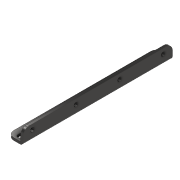
# Autodesk Inventor part: beugel armsteun
Saved by Autodesk Inventor 2020.3 (Build 243373000, 373)
## iProperties
Created: 2020-09-11
Part Number: beugel armsteun
Material: Stainless Steel
Document SubType Name: Modeling
Designer: Svend
Density: 8 g/cm^3
Appearance: Semi-Polished
Author: Svend
Autodesk Inventor part; units mm, degrees
ref_plane "YZ Plane" through (0, 0, 0) normal (1, 0, 0) x (0, 1, 0)
ref_plane "XZ Plane" through (0, 0, 0) normal (0, 1, 0) x (-1, 0, 0)
ref_plane "XY Plane" through (0, 0, 0) normal (0, 0, 1) x (1, 0, 0)
sketch "Sketch1" plane through (0, 0, 0) normal (0, 0, 1) x (1, 0, 0)
  line L0 (0, 0) -> (-25, 0)
  line L1 (-25, 0) -> (-25, 4)
  line L2 (-25, 4) -> (-4, 4)
  line L3 (-4, 4) -> (-4, 23)
  line L4 (-4, 23) -> (0, 23)
  line L5 (0, 23) -> (0, 0)
  dimension "d0" = 25
  dimension "d1" = 4
  dimension "d2" = 23
  constraints: 12 end point, 4 perpendicular, 3 horizontal
  measures "d0" distance of L0.start L0.end
  measures "d1" distance of L0.end L1.end
  measures "d2" distance of L4.end L0.start
extrude "Extrusion1" add sketch "Sketch1" along normal mid plane 240
sketch "Sketch2" plane through (-4, 4, 120) normal (-1, 0, 0) x (0, 0, 1)
  circle A0 centre (-225, 11) radius 3.5
  line L0 (-240, 0) -> (-240, 19) projected
  line L1 (-240, 19) -> (0, 19) projected
  circle A1 centre (-155, 11) radius 3.5
  circle A2 centre (-85, 11) radius 3.5
  circle A3 centre (-15, 11) radius 3.5
  line L2 (0, 19) -> (0, 0) projected
  point P0 (-120, -4)
  dimension "d5" = 7
  dimension "d6" = 15
  dimension "d7" = 8
  dimension "d8" = 15
  dimension "d9" = 70
  dimension "d10" = 70
  constraints: 4 centre point, 3 equal radius, 3 horizontal alignment
  measures "d5" diameter of A0
  measures "d6" distance from line of L0 A0.centre
  measures "d7" distance from line of A0.centre L1
  measures "d8" distance from line of L2 A3.centre
  measures "d9" distance of A2.centre A3.centre
  measures "d10" distance of A0.centre A1.centre
extrude "Extrusion2" cut sketch "Sketch2" against normal blind 10
sketch "Sketch3" plane through (-25, 4, 120) normal (0, 1, 0) x (1, 0, 0)
  circle A0 centre (12.5, 7) radius 3.5
  line L0 (0, 240) -> (0, 0) projected
  line L1 (21, 0) -> (0, 0) projected
  circle A1 centre (12.5, 45) radius 3.5
  line L2 (16, 45) -> (16, 7)
  line L3 (9, 7) -> (9, 45)
  line L4 (21, 240) -> (21, 0) construction
  line L5 (21, 120) -> (0, 120) construction
  circle A2 centre (12.5, 233) radius 3.5
  circle A3 centre (12.5, 195) radius 3.5
  line L6 (16, 195) -> (16, 233)
  line L7 (9, 233) -> (9, 195)
  point P0 (25, 120)
  dimension "d13" = 7
  dimension "d14" = 12.5
  dimension "d15" = 7
  dimension "d16" = 38
  constraints: 10 end point, 8 point on circle, 6 symmetric about line, 4 centre point, 4 tangent, 2 midpoint, 1 equal radius, 1 vertical alignment, 2 other
  measures "d13" diameter of A0
  measures "d14" distance from line of L0 A0.centre
  measures "d15" distance from line of L1 A0.centre
  measures "d16" distance of A1.centre A0.centre
extrude "Extrusion3" cut sketch "Sketch3" against normal blind 10
fillet "Fillet1" radius 5 1 edges at (0, 0, 0)
fillet "Fillet2" radius 10 4 edges at (-2, 23, -120) (-25, 2, -120) (-25, 2, 120) (-2, 23, 120)
equation "\"d8\" = d6"
equation "\"d10\" = d9"
body "Solid1"
